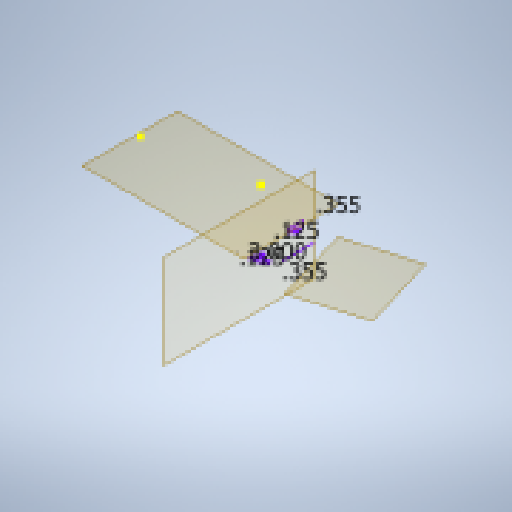
# Autodesk Inventor part: WashChamberConduit
Saved by Autodesk Inventor 2024 (Build 280153000, 153)
## iProperties
Created: 2024-09-07
Part Number: WashChamberConduit
Material: Generic
Document SubType Name: Modeling
Designer: Tommy Rohmann
Density: 1 g/cm^3
Appearance: Default
Author: Tommy Rohmann
Autodesk Inventor part; units mm, degrees
ref_plane "YZ Plane" through (0, 0, 0) normal (1, 0, 0) x (0, 1, 0)
ref_plane "XZ Plane" through (0, 0, 0) normal (0, 1, 0) x (-1, 0, 0)
ref_plane "XY Plane" through (0, 0, 0) normal (0, 0, 1) x (1, 0, 0)
sketch "Sketch5" plane through (0, 0, 0) normal (0, 1, 0) x (-1, 0, 0)
  line L0 (-272.8857, 16.2919) -> (-285.5857, 16.2919)
  line L1 (-285.5857, 16.2919) -> (-285.5857, 21.0544)
  line L2 (-285.5857, 21.0544) -> (-280.6644, 21.0544)
  line L3 (-280.6644, 26.3249) -> (-285.5857, 26.3249)
  line L4 (-280.6644, 21.0544) -> (-280.6644, 26.3249)
  line L5 (-280.6644, 31.0874) -> (-285.5857, 31.0874)
  line L6 (-285.5857, 26.3249) -> (-285.5857, 31.0874)
  line L7 (-280.6644, 31.0874) -> (-280.6644, 36.3579)
  line L8 (-285.5857, 36.3579) -> (-285.5857, 41.1204)
  line L9 (-285.5857, 41.1204) -> (-266.3769, 41.1204)
  line L10 (-272.8857, 9.9419) -> (-272.8857, 16.2919)
  line L11 (-266.3769, -18.3156) -> (-266.3769, 41.1204)
  line L12 (-291.7769, 9.9419) -> (-272.8857, 9.9419)
  line L13 (-282.7599, -18.3156) -> (-266.3769, -18.3156)
  line L14 (-291.7769, 6.7669) -> (-282.7599, -18.3156)
  line L15 (-291.7769, 6.7669) -> (-291.7769, 9.9419)
  line L16 (-280.6644, 36.3579) -> (-285.5857, 36.3579)
  line L17 (-342.5769, -58.268) -> (-342.5769, 69.8263)
  line L18 (-266.3769, -0.8164) -> (-269.5519, -0.8164)
  line L19 (-269.5519, -0.8164) -> (-269.5519, 2.3586)
  line L20 (-269.5519, 2.3586) -> (-266.3769, 2.3586)
  point P0 (0, 0)
  dimension "d34" = 3.175
  dimension "d35" = 9.017
  dimension "d36" = 50.8
  dimension "d37" = 76.2
  dimension "d39" = 61.9125
  dimension "d40" = 6.35
  dimension "d41" = 56.9913
  dimension "d42" = 12.7
  dimension "d43" = 3.175
  dimension "d44" = 3.175
  dimension "d45" = 17.4992
  dimension "d46" = 28.2575
  dimension "d47" = 4.7625
  constraints: 42 end point, 8 horizontal, 5 collinear, 3 perpendicular, 2 point on line, 1 vertical
  measures "d34" distance of L15.start L15.end
  measures "d35" horizontal distance of L14.end L15.start
  measures "d36" distance between parallel lines of L15 L17
  measures "d37" distance between parallel lines of L17 L11
  measures "d39" distance between parallel lines of L17 L4
  measures "d40" distance of L12.end L0.start
  measures "d41" distance between parallel lines of L17 L8
  measures "d42" distance of L0.start L1.start
  measures "d43" distance of L19.end L20.end
  measures "d44" distance of L18.end L19.end
  measures "d45" distance between parallel lines of L13 L18
  measures "d46" distance between parallel lines of L13 L12
  measures "d47" distance of L1.start L1.end
revolve "Revolution2" add sketch "Sketch5" angle 360 about axis through (342.5769, 0, -58.268) along (0, 0, 1) contours L0 L1 L2 L4 L3 L6 L5 L7 L16 L8 L9 L11 L20 L19 L18 L13 L14 L15 L12 L10
equation "\"d41\" = 0.5 * WashChamberOD - SealedSurfaceOffset"
equation "\"d47\" = StaticORingThickness"
equation "\"MachineMaxHeight\" = 539.75"
equation "\"MachineMaxWidth\" = 215.9"
equation "\"MachineMaxLength\" = 266.7"
equation "\"MachineFluidCapacity\" = 25.4"
equation "\"MaxCompressiveCapacity\" = 20320"
equation "\"WashChamberID\" = 101.6"
equation "\"WashChamberOD\" = 114.3"
equation "\"ConduitThickness\" = 152.4"
equation "\"StaticORingThickness\" = 4.7625"
equation "\"SealedSurfaceOffset\" = 0.15875"
body "Solid2"
